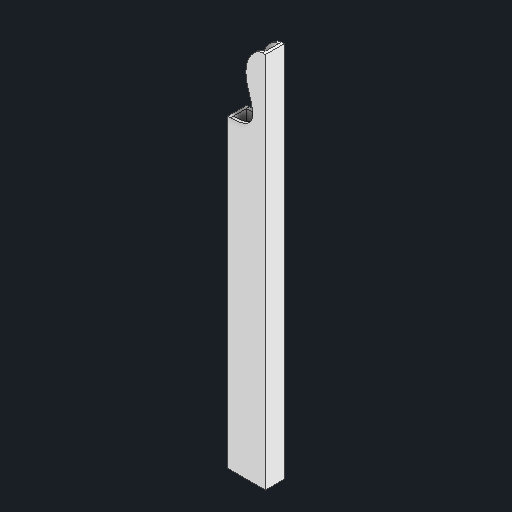
# Autodesk Inventor part: tibea_profile
Saved by Autodesk Inventor 2026 (Build 300175000, 175)
## iProperties
Created: 2026-04-23
Part Number: tibea_profile
Material: Алюминий
Document SubType Name: Modeling
Designer: user
Density: 2.7 g/cm^3
Appearance: Белый
Mass: 312.742 g
Surface Area: 782.849 cm^2
Volume: 115.83 cm^3
Author: user
Autodesk Inventor part; units mm, degrees
ref_plane "YZ Plane" through (0, 0, 0) normal (1, 0, 0) x (0, 1, 0)
ref_plane "XZ Plane" through (0, 0, 0) normal (0, 1, 0) x (-1, 0, 0)
ref_plane "XY Plane" through (0, 0, 0) normal (0, 0, 1) x (1, 0, 0)
sketch "Эскиз1" plane through (0, 0, 0) normal (0, 1, 0) x (-1, 0, 0)
  line L0 (0, 0) -> (40, 0)
  line L1 (40, 0) -> (40, -20)
  line L2 (40, -20) -> (0, -20)
  line L3 (0, -20) -> (0, 0)
  line L4 (37, -3) -> (3, -3)
  line L5 (3, -3) -> (3, -17)
  line L6 (3, -17) -> (37, -17)
  line L7 (37, -17) -> (37, -3)
  dimension "d0" = 20
  dimension "d1" = 40
  dimension "d2" = 3
  constraints: 16 end point, 4 parallel, 2 perpendicular, 1 horizontal, 3 other
  measures "d0" distance of L0.end L1.end
  measures "d1" distance of L1.end L2.end
  measures "d2" distance between parallel lines of L0 L4
extrude "Выдавливание1" add sketch "Эскиз1" along normal blind 400
sketch "Эскиз2" plane through (-40, 0, 0) normal (0, 0, 1) x (1, 0, 0)
  line L0 (3, 0) -> (3, 400) projected
  line L1 (0, 400) -> (40, 400) projected
  line L2 (20, 819.3664) -> (20, 691.613)
  line L3 (3, 0) -> (37, 0) projected
  line L4 (37, 0) -> (37, 400) projected
  line L5 (3, 400) -> (37, 400) projected
  line L6 (3, 0) -> (3, 400) projected
  line L7 (37, 0) -> (37, 400) projected
  spline S0 degree 4 poles (37, 400) (28.1429, 400) (6.6723, 373.0542) (29.5104, 351.5723) (31.0092, 323.4583) (3, 323.4583) knots 0 0 0 0 0 0.490634 1 1 1 1 1
  line L8 (22.2784, 323.4583) -> (-16.2784, 323.4583) construction
  arc A0 (-12.0901, 325.0339) -> (18.0901, 325.0339) centre (3, 396.5064) ccw construction
  line L9 (44.0036, 400) -> (29.9964, 400) construction
  arc A1 (41.5725, 398.5449) -> (32.4275, 398.5449) centre (37, 392.0879) ccw construction
  line L10 (3, 323.4583) -> (0, 323.4583)
  line L11 (0, 0) -> (0, 400) projected
  line L12 (0, 323.4583) -> (0, 400)
  point P0 (40, 0)
  point P1 (20, 381.1712)
  point P2 (25.6195, 346.1519)
  constraints: 10 end point, 4 midpoint, 3 horizontal, 2 centre point, 2 perpendicular, 2 point on circle, 1 parallel, 1 point on line, 1 vertical, 6 other
extrude "Выдавливание2" cut sketch "Эскиз2" against normal through all contours L10 L11 L1 L0 | L0 L1 S0
equation "\"d0\" = width_profile_tibea"
equation "\"d1\" = hight_profile_tibea"
equation "\"d2\" = thickness_profile_tibea"
equation "\"d3\" = length_thorn_tibia"
equation "\"d_main_shaft\" = 15"
equation "\"width_profile_tibea\" = 20"
equation "\"hight_profile_tibea\" = 40"
equation "\"thickness_profile_tibea\" = 3"
equation "\"tolerance_plazma\" = 0.1"
equation "\"d_main_screw_holes\" = 6.1"
equation "\"length_thorn_tibia\" = 400"
equation "\"thickness_steel\" = 3"
equation "\"hight_shaft_shift\" = 37"
equation "\"thickness_profile_femur\" = 3"
equation "\"width_shaft_shift\" = 35"
equation "\"width_flattened_surface\" = 12"
